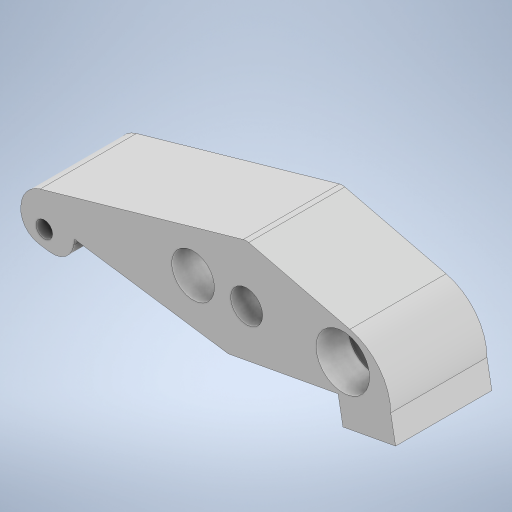
# Autodesk Inventor part: Bauteil2
Saved by Autodesk Inventor 2023 (Build 270158000, 158)
## iProperties
Created: 2024-02-02
Part Number: Bauteil2
Material: Generisch
Document SubType Name: Modeling
Designer: jefar
Density: 1 g/cm^3
Appearance: Vorgabe
Author: jefar
Autodesk Inventor part; units mm, degrees
ref_plane "YZ Plane" through (0, 0, 0) normal (1, 0, 0) x (0, 1, 0)
ref_plane "XZ Plane" through (0, 0, 0) normal (0, 1, 0) x (-1, 0, 0)
ref_plane "XY Plane" through (0, 0, 0) normal (0, 0, 1) x (1, 0, 0)
sketch "Skizze1" plane through (0, 0, 0) normal (0, 0, 1) x (1, 0, 0)
  arc A0 (3118.8287, 148.9752) -> (2736.7523, 634.8703) centre (2618.8287, 148.9752) ccw
  line L0 (2736.7523, 634.8703) -> (1790.5787, 864.5036)
  line L1 (1739.6109, 863.5025) -> (-158.5948, 323.0655)
  arc A1 (-158.5948, 323.0655) -> (-331.1713, 148.9752) centre (-90.1379, 82.6208) ccw
  arc A2 (1765.4752, 870.5961) -> (1764.4558, 870.5761) centre (1765.0035, 868.6526) ccw
  arc A3 (1790.5787, 864.5036) -> (1739.6109, 863.5025) centre (1766.9937, 767.3247) ccw
  line L2 (-331.1713, 148.9752) -> (1600.5878, -131.3474)
  line L3 (1600.5878, -131.3474) -> (3118.8287, 148.9752)
  point P0 (0, 0)
  point P1 (1764.9629, 870.7205)
  dimension "d1" = 1000
  dimension "d2" = 2000
  dimension "d3" = 500
  dimension "d4" = 250
  constraints: 8 end point, 8 point on circle, 5 tangent, 4 centre point, 4 point on line
  measures "d1" distance of L0.start point (1764.963, 870.72)
  measures "d2" distance of point (1764.963, 870.72) L1.end
  measures "d3" radius of A0
  measures "d4" radius of A1
extrude "Extrusion1" add sketch "Skizze1" along normal blind 900
sketch "Skizze2" plane through (3118.8287, 148.9752, 0) normal (0.1815675, -0.9833785, 0) x (0.9833785, 0.1815675, 0)
  line L0 (-1543.9029, 900) -> (0, 900) construction
  line L1 (-1543.9029, 0) -> (0, 0) construction
  line L2 (0, 900) -> (-500, 900)
  line L3 (-500, 900) -> (-500, 0)
  line L4 (-500, 0) -> (0, 0)
  line L5 (0, 0) -> (0, 900)
  line L6 (-3191.3386, 900) -> (-3392.6558, 900) projected
  line L7 (-1226.5582, 0) -> (-3191.3386, 0) construction
  line L8 (-3392.6558, 900) -> (-2892.6558, 900)
  line L9 (-2892.6558, 900) -> (-2892.6558, 0)
  line L10 (-2892.6558, 0) -> (-3392.6558, 0)
  line L11 (-3392.6558, 0) -> (-3392.6558, 900)
  point P0 (-3094.0381, 0)
  dimension "d16" = 500
  dimension "d17" = 500
  constraints: 16 end point, 4 parallel, 2 horizontal, 2 perpendicular, 2 point on line
  measures "d16" distance of L4.end L3.end
  measures "d17" distance of L9.end L10.end
extrude "Extrusion2" add sketch "Skizze2" along normal blind 250 contours L5 L4 L3 L2
sketch "Skizze3" plane through (1600.5878, -131.3474, 0) normal (-0.1436085, -0.9896346, 0) x (0.9896346, -0.1436085, 0)
  line L0 (-1951.9923, 0) -> (0, 0) construction
  line L1 (-1951.9923, 900) -> (0, 900) construction
  line L2 (-1951.9923, 0) -> (-1451.9923, 0)
  line L3 (-1451.9923, 0) -> (-1451.9923, 900)
  line L4 (-1451.9923, 900) -> (-1951.9923, 900)
  line L5 (-1951.9923, 900) -> (-1951.9923, 0)
  point P0 (-1602.8597, 0)
  dimension "d20" = 500
  constraints: 8 end point, 2 parallel, 1 horizontal, 1 perpendicular, 1 point on line
  measures "d20" distance of L4.end L3.end
extrude "Extrusion3" add sketch "Skizze3" along normal blind 250
sketch "Skizze4" plane through (-331.1713, 148.9752, 0) normal (-0.9896346, 0.1436085, 0) x (0, 0, 1)
  line L0 (0, 0) -> (0, 197.0692) construction
  line L1 (900, 0) -> (900, -250) projected
  line L2 (0, 0) -> (900, 0)
  line L3 (900, 0) -> (900, -250)
  line L4 (900, -250) -> (0, -250)
  line L5 (0, -250) -> (0, 0)
  point P0 (0, -99.872)
  constraints: 8 end point, 2 parallel, 1 horizontal, 1 perpendicular
sketch "Skizze5" plane through (0, 0, 900) normal (0, 0, 1) x (1, 0, 0)
  line L0 (163.646, 77.171) -> (1600.5878, -131.3474) construction
  line L1 (1600.5878, -131.3474) -> (2100.5878, -131.3474) construction
  circle A0 centre (1771.5979, 338.4989) radius 150
  point P0 (0, 0)
  dimension "d25" = 300
  constraints: 2 end point, 1 centre point, 1 horizontal
  measures "d25" diameter of A0
extrude "Extrusion4" cut sketch "Skizze5" against normal through all
sketch "Skizze6" plane through (0, 0, 900) normal (0, 0, 1) x (1, 0, 0)
  circle A0 centre (-119.6648, 15.6644) radius 77.6159
  point P0 (0, 0)
  constraints: 1 centre point
extrude "Extrusion5" cut sketch "Skizze6" against normal through all
sketch "Skizze7" plane through (-331.1713, 148.9752, 0) normal (-0.9896346, 0.1436085, 0) x (0, 0, 1)
  point P0 (0, -99.872)
sketch "Skizze8" plane through (-331.1713, 148.9752, 0) normal (-0.9896346, 0.1436085, 0) x (0, 0, 1)
  line L0 (900, 0) -> (0, 0) construction
  line L1 (0, -250) -> (900, -250) construction
  line L2 (450, 0) -> (600, 0)
  line L3 (600, 0) -> (600, -250)
  line L4 (600, -250) -> (450, -250)
  line L5 (450, -250) -> (450, 0)
  line L6 (450, 0) -> (300, 0)
  line L7 (300, 0) -> (300, -250)
  line L8 (300, -250) -> (450, -250)
  line L9 (450, -250) -> (450, 0)
  point P0 (0, -99.872)
  dimension "d31" = 150
  dimension "d32" = 150
  constraints: 16 end point, 4 parallel, 2 horizontal, 2 perpendicular, 2 point on line, 1 midpoint
  measures "d31" distance of L3.end L4.end
  measures "d32" distance of L8.end L7.end
extrude "Extrusion6" cut sketch "Skizze8" against normal through all
fillet "Rundung1" radius 200 4 edges at (-367.0734, -98.4335, 750) (-367.0734, -98.4335, 150) (127.7439, -170.2377, 150) (127.7439, -170.2377, 750)
sketch "Skizze9" plane through (0, 0, 900) normal (0, 0, 1) x (1, 0, 0)
  circle A0 centre (1271.5979, 338.4989) radius 200
  point P0 (0, 0)
  dimension "d37" = 400
  constraints: 1 centre point
  measures "d37" diameter of A0
extrude "Extrusion7" cut sketch "Skizze9" against normal blind 300
sketch "Skizze10" plane through (0, 0, 900) normal (0, 0, 1) x (1, 0, 0)
  circle A0 centre (2671.5979, 338.4989) radius 250
  point P0 (0, 0)
  dimension "d41" = 500
  constraints: 1 centre point
  measures "d41" diameter of A0
extrude "Extrusion8" cut sketch "Skizze10" against normal blind 300
